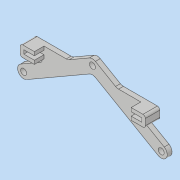
# Autodesk Inventor part: ServoControllerHolder
Saved by Autodesk Inventor 2017 (Build 210142000, 142)
## iProperties
Created: 2017-04-24
Part Number: ServoControllerHolder
Material: Generic
Document SubType Name: Modeling
Designer: Derek Wider
Mass: 2.15654 g
Surface Area: 24.5428 cm^2
Volume: 2.15654 cm^3
Density: 1 g/cm^3
Appearance: Default
Author: Derek Wider
Autodesk Inventor part; units mm, degrees
ref_plane "YZ Plane" through (0, 0, 0) normal (1, 0, 0) x (0, 1, 0)
ref_plane "XZ Plane" through (0, 0, 0) normal (0, 1, 0) x (-1, 0, 0)
ref_plane "XY Plane" through (0, 0, 0) normal (0, 0, 1) x (1, 0, 0)
sketch "Sketch2" plane through (0, 0, 0) normal (0, 0, 1) x (1, 0, 0)
  circle A0 centre (0, 0) radius 1.5875
  circle A1 centre (0, 0) radius 3.175
  line L0 (0, 0) -> (36.2951, 20.955)
  line L1 (0, 0) -> (41.91, 0) construction
  line L2 (36.2951, 20.955) -> (72.5902, 0)
  circle A2 centre (72.5902, 0) radius 1.5875
  circle A3 centre (72.5902, 0) radius 3.175
  circle A4 centre (36.2951, 20.955) radius 1.5875
  circle A5 centre (36.2951, 20.955) radius 3.175
  line L3 (-1.5875, 2.7496) -> (34.7076, 23.7046)
  line L4 (74.1777, 2.7496) -> (37.8826, 23.7046)
  line L5 (71.0027, -2.7496) -> (36.2951, 17.2888)
  line L6 (36.2951, 17.2888) -> (1.5875, -2.7496)
  line L7 (36.2951, 20.955) -> (36.2951, 17.145)
  line L8 (67.4101, 15.24) -> (5.1801, 15.24)
  line L9 (5.1801, 15.24) -> (5.1801, 17.145)
  line L10 (5.1801, 17.145) -> (67.4101, 17.145)
  line L11 (67.4101, 17.145) -> (67.4101, 15.24)
  line L12 (5.1801, 13.208) -> (67.4101, 13.208)
  line L13 (67.4101, 13.208) -> (67.4101, 11.303)
  line L14 (67.4101, 11.303) -> (5.1801, 11.303)
  line L15 (5.1801, 11.303) -> (5.1801, 13.208)
  line L16 (10.7681, 17.145) -> (61.8221, 17.145)
  line L17 (61.8221, 17.145) -> (61.8221, 11.303)
  line L18 (61.8221, 11.303) -> (10.7681, 11.303)
  line L19 (10.7681, 11.303) -> (10.7681, 17.145)
  line L20 (10.7681, 17.145) -> (61.8221, 17.145)
  line L21 (61.8221, 17.145) -> (61.8221, 11.303)
  line L22 (61.8221, 11.303) -> (10.7681, 11.303)
  line L23 (10.7681, 11.303) -> (10.7681, 17.145)
  line L24 (5.1801, 17.145) -> (3.2751, 17.145)
  line L25 (3.2751, 17.145) -> (3.2751, 11.303)
  line L26 (3.2751, 11.303) -> (5.1801, 11.303)
  line L27 (5.1801, 11.303) -> (5.1801, 17.145)
  line L28 (67.4101, 11.303) -> (69.3151, 11.303)
  line L29 (69.3151, 11.303) -> (69.3151, 17.145)
  line L30 (69.3151, 17.145) -> (67.4101, 17.145)
  line L31 (67.4101, 17.145) -> (67.4101, 11.303)
  dimension "d5" = 3.175
  dimension "d6" = 6.35
  dimension "d7" = 41.91
  dimension "d8" = 30
  dimension "d9" = 41.91
  dimension "d10" = 120
  dimension "d11" = 3.175
  dimension "d12" = 6.35
  dimension "d13" = 3.175
  dimension "d14" = 6.35
  dimension "d15" = 3.81
  dimension "d16" = 62.23
  dimension "d17" = 31.115
  dimension "d18" = 2.032
  dimension "d19" = 1.905
  dimension "d20" = 1.905
  dimension "d21" = 5.588
  dimension "d22" = 5.588
  dimension "d23" = 1.905
  dimension "d24" = 1.905
  constraints: 64 end point, 14 parallel, 7 horizontal, 6 centre point, 6 coincident, 6 perpendicular, 6 point on circle, 3 point on line, 3 tangent, 2 vertical alignment, 1 equal length, 1 midpoint, 1 vertical
  measures "d5" diameter of A0
  measures "d6" diameter of A1
  measures "d7" distance of L0.start L0.end
  measures "d8" angle of L1 L0
  measures "d9" distance of L0.end L2.end
  measures "d10" angle of L0 L2
  measures "d11" diameter of A2
  measures "d12" diameter of A3
  measures "d13" diameter of A4
  measures "d14" diameter of A5
  measures "d15" distance of L7.start L7.end
  measures "d16" distance of L9.end L10.end
  measures "d17" distance between parallel lines of L7 L11
  measures "d18" distance between parallel lines of L8 L12
  measures "d19" distance of L8.end L9.end
  measures "d20" distance of L14.end L12.start
  measures "d21" distance between parallel lines of L19 L9
  measures "d22" distance between parallel lines of L11 L17
  measures "d23" distance of L26.end L25.end
  measures "d24" distance of L30.end L29.end
extrude "Extrusion1" add sketch "Sketch2" along normal blind 2.54 contours A1 | L3 L14 L0 A1 | A1 L0 L14 L6 | L14 L19 L12 L3 | L3 L12 L0 L14 | L14 L0 L12 L6 | L6 L12 L5 L14 | L3 L8 L0 L12 | L14 L15 L12 L19 | L12 L0 L8 L6 | L14 L2 A3 L5 | L5 L12 L2 L14 | L8 L19 L10 L3 | L3 L10 L0 L8 | L26 L25 L24 L9 L27 L15 | L8 L0 L10 L6 | L6 L10 L5 L8 | L5 L8 L2 L12 | A3 | L14 L4 A3 L2 | L2 L12 L4 L14 | L3 A5 L0 L10 | L8 L9 L10 L19 | L10 L0 A5 L7 L6 | L5 L10 L2 L8 | L2 L8 L4 L12 | L4 L12 L17 L14 | A5 L2 A4 L0 | L7 A5 L2 L10 L5 | L2 L10 L4 L8 | L17 L12 L13 L14 | L0 A4 L7 A5 | L4 L10 L2 A5 | L7 A4 L2 A5 | L4 L10 L17 L8 | L13 L31 L11 L30 L29 L28 | L17 L10 L11 L8
sketch "Sketch4" plane through (0, 0, 2.54) normal (0, 0, 1) x (1, 0, 0)
  line L0 (69.3151, 17.145) -> (49.2442, 17.145) projected
  line L1 (49.2442, 17.145) -> (37.8826, 23.7046) projected
  arc A0 (37.8826, 23.7046) -> (34.7076, 23.7046) centre (36.2951, 20.955) ccw projected
  line L2 (34.7076, 23.7046) -> (23.346, 17.145) projected
  line L3 (23.346, 17.145) -> (3.2751, 17.145) projected
  line L4 (3.2751, 17.145) -> (3.2751, 11.303) projected
  line L5 (3.2751, 11.303) -> (13.2274, 11.303) projected
  line L6 (13.2274, 11.303) -> (-1.5875, 2.7496) projected
  arc A1 (-1.5875, 2.7496) -> (1.5875, -2.7496) centre (0, 0) ccw projected
  line L7 (1.5875, -2.7496) -> (25.9274, 11.303) projected
  line L8 (25.9274, 11.303) -> (46.6629, 11.303) projected
  line L9 (46.6629, 11.303) -> (71.0027, -2.7496) projected
  arc A2 (71.0027, -2.7496) -> (74.1777, 2.7496) centre (72.5902, 0) ccw projected
  line L10 (74.1777, 2.7496) -> (59.3629, 11.303) projected
  line L11 (59.3629, 11.303) -> (69.3151, 11.303) projected
  line L12 (69.3151, 11.303) -> (69.3151, 17.145) projected
  line L13 (5.1801, 15.24) -> (20.0465, 15.24) projected
  line L14 (20.0465, 15.24) -> (16.5269, 13.208) projected
  line L15 (16.5269, 13.208) -> (5.1801, 13.208) projected
  line L16 (5.1801, 13.208) -> (5.1801, 15.24) projected
  line L17 (36.046, 17.145) -> (36.2951, 17.2888) projected
  line L18 (36.2951, 17.2888) -> (36.5442, 17.145) projected
  line L19 (36.5442, 17.145) -> (36.046, 17.145) projected
  line L20 (67.4101, 15.24) -> (67.4101, 13.208) projected
  line L21 (67.4101, 13.208) -> (56.0633, 13.208) projected
  line L22 (56.0633, 13.208) -> (52.5438, 15.24) projected
  line L23 (52.5438, 15.24) -> (67.4101, 15.24) projected
  circle A3 centre (36.2951, 20.955) radius 1.5875 projected
  circle A4 centre (0, 0) radius 1.5875 projected
  circle A5 centre (72.5902, 0) radius 1.5875 projected
  line L24 (32.7465, 15.24) -> (39.8438, 15.24) projected
  line L25 (39.8438, 15.24) -> (43.3633, 13.208) projected
  line L26 (43.3633, 13.208) -> (29.2269, 13.208) projected
  line L27 (29.2269, 13.208) -> (32.7465, 15.24) projected
  line L28 (10.7681, 17.145) -> (10.7681, 15.24)
  line L29 (10.7681, 13.208) -> (10.7681, 11.303)
  line L30 (61.8221, 17.145) -> (61.8221, 15.24)
  line L31 (61.8221, 13.208) -> (61.8221, 11.303)
  constraints: 10 point on line, 8 end point, 2 perpendicular
extrude "Extrusion2" add sketch "Sketch4" along normal blind 5.08 contours L12 L11 L31 L21 L20 L23 L30 L0 | L28 L13 L16 L15 L29 L5 L4 L3
sketch "Sketch5" plane through (0, 0, 0) normal (0, 0, -1) x (-1, 0, 0)
  line L0 (-67.4101, 15.24) -> (-67.4101, 13.208) projected
  line L1 (-52.5438, 15.24) -> (-67.4101, 15.24) projected
  line L2 (-56.0633, 13.208) -> (-52.5438, 15.24) projected
  line L3 (-67.4101, 13.208) -> (-56.0633, 13.208) projected
  circle A0 centre (-72.5902, 0) radius 1.5875 projected
  circle A1 centre (-36.2951, 20.955) radius 1.5875 projected
  circle A2 centre (0, 0) radius 1.5875 projected
  line L4 (-32.7465, 15.24) -> (-39.8438, 15.24) projected
  line L5 (-29.2269, 13.208) -> (-32.7465, 15.24) projected
  line L6 (-43.3633, 13.208) -> (-29.2269, 13.208) projected
  line L7 (-39.8438, 15.24) -> (-43.3633, 13.208) projected
  line L8 (-5.1801, 13.208) -> (-5.1801, 15.24) projected
  line L9 (-16.5269, 13.208) -> (-5.1801, 13.208) projected
  line L10 (-20.0465, 15.24) -> (-16.5269, 13.208) projected
  line L11 (-5.1801, 15.24) -> (-20.0465, 15.24) projected
  line L12 (-36.2951, 17.2888) -> (-36.5442, 17.145) projected
  line L13 (-36.046, 17.145) -> (-36.2951, 17.2888) projected
  line L14 (-36.5442, 17.145) -> (-36.046, 17.145) projected
  line L15 (-59.3629, 11.303) -> (-69.3151, 11.303) projected
  line L16 (-74.1777, 2.7496) -> (-59.3629, 11.303) projected
  arc A3 (-74.1777, 2.7496) -> (-71.0027, -2.7496) centre (-72.5902, 0) ccw projected
  line L17 (-46.6629, 11.303) -> (-71.0027, -2.7496) projected
  line L18 (-25.9274, 11.303) -> (-46.6629, 11.303) projected
  line L19 (-1.5875, -2.7496) -> (-25.9274, 11.303) projected
  arc A4 (-1.5875, -2.7496) -> (1.5875, 2.7496) centre (0, 0) ccw projected
  line L20 (-13.2274, 11.303) -> (1.5875, 2.7496) projected
  line L21 (-3.2751, 11.303) -> (-13.2274, 11.303) projected
  line L22 (-3.2751, 17.145) -> (-3.2751, 11.303) projected
  line L23 (-23.346, 17.145) -> (-3.2751, 17.145) projected
  line L24 (-34.7076, 23.7046) -> (-23.346, 17.145) projected
  arc A5 (-34.7076, 23.7046) -> (-37.8826, 23.7046) centre (-36.2951, 20.955) ccw projected
  line L25 (-49.2442, 17.145) -> (-37.8826, 23.7046) projected
  line L26 (-69.3151, 17.145) -> (-49.2442, 17.145) projected
  line L27 (-69.3151, 11.303) -> (-69.3151, 17.145) projected
  line L28 (-46.6629, 11.303) -> (-36.2951, 17.2888)
  line L29 (-36.2951, 17.2888) -> (-25.9274, 11.303)
  line L30 (-46.6629, 11.303) -> (-25.9274, 11.303)
  constraints: 6 end point, 2 collinear
extrude "Extrusion3" cut sketch "Sketch5" against normal blind 5.08 contours L4 L28 L14 L29 | L29 L18 L28 L6
sketch "Sketch6" plane through (0, 0, 0) normal (0, 0, -1) x (-1, 0, 0)
  line L0 (-5.1801, 13.208) -> (-5.1801, 15.24) projected
  line L1 (-16.5269, 13.208) -> (-5.1801, 13.208) projected
  line L2 (-20.0465, 15.24) -> (-16.5269, 13.208) projected
  line L3 (-5.1801, 15.24) -> (-20.0465, 15.24) projected
  circle A0 centre (0, 0) radius 1.5875 projected
  circle A1 centre (-36.2951, 20.955) radius 1.5875 projected
  circle A2 centre (-72.5902, 0) radius 1.5875 projected
  line L4 (-67.4101, 15.24) -> (-67.4101, 13.208) projected
  line L5 (-52.5438, 15.24) -> (-67.4101, 15.24) projected
  line L6 (-56.0633, 13.208) -> (-52.5438, 15.24) projected
  line L7 (-67.4101, 13.208) -> (-56.0633, 13.208) projected
  line L8 (-71.0027, -2.7496) -> (-36.2951, 17.2888) projected
  line L9 (-36.2951, 17.2888) -> (-1.5875, -2.7496) projected
  arc A3 (-1.5875, -2.7496) -> (1.5875, 2.7496) centre (0, 0) ccw projected
  line L10 (-13.2274, 11.303) -> (1.5875, 2.7496) projected
  line L11 (-3.2751, 11.303) -> (-13.2274, 11.303) projected
  line L12 (-3.2751, 17.145) -> (-3.2751, 11.303) projected
  line L13 (-23.346, 17.145) -> (-3.2751, 17.145) projected
  line L14 (-34.7076, 23.7046) -> (-23.346, 17.145) projected
  arc A4 (-34.7076, 23.7046) -> (-37.8826, 23.7046) centre (-36.2951, 20.955) ccw projected
  line L15 (-49.2442, 17.145) -> (-37.8826, 23.7046) projected
  line L16 (-69.3151, 17.145) -> (-49.2442, 17.145) projected
  line L17 (-69.3151, 11.303) -> (-69.3151, 17.145) projected
  line L18 (-59.3629, 11.303) -> (-69.3151, 11.303) projected
  line L19 (-74.1777, 2.7496) -> (-59.3629, 11.303) projected
  arc A5 (-74.1777, 2.7496) -> (-71.0027, -2.7496) centre (-72.5902, 0) ccw projected
extrude "Extrusion4" add sketch "Sketch6" against normal up to surface (2.54 mm away) contours L1 L2 L3 L0 | L5 L6 L7 L4
fillet "Fillet1" radius 3.175 3 edges at (36.2951, 17.2888, 1.27) (23.346, 17.145, 1.27) (49.2442, 17.145, 1.27)
fillet "Fillet2" radius 1.27 6 edges at (59.3629, 11.303, 1.27) (69.3151, 11.303, 3.81) (69.3151, 17.145, 3.81) (3.2751, 11.303, 3.81) (3.2751, 17.145, 3.81) (13.2274, 11.303, 1.27)
equation "\"d17\" = 0.5 * d16"
equation "\"d22\" = d21"
body "Solid1"
